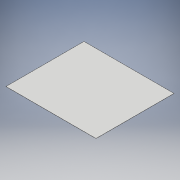
# Autodesk Inventor part: leftPanel
Saved by Autodesk Inventor 2017 (Build 210142000, 142)
## iProperties
Created: 2017-06-07
Part Number: leftPanel
Material: Generic
Document SubType Name: Sheet Metal
Designer: Roko
Density: 1 g/cm^3
Sheet Metal Rule: Default_mm
Appearance: Default
Author: Roko
Autodesk Inventor part; units mm, degrees
ref_plane "YZ Plane" through (0, 0, 0) normal (1, 0, 0) x (0, 1, 0)
ref_plane "XZ Plane" through (0, 0, 0) normal (0, 1, 0) x (-1, 0, 0)
ref_plane "XY Plane" through (0, 0, 0) normal (0, 0, 1) x (1, 0, 0)
sketch "Sketch1" plane through (0, 0, 0) normal (0, 0, 1) x (1, 0, 0)
  line L0 (-150, -130) -> (150, -130)
  line L1 (150, -130) -> (150, 130)
  line L2 (150, 130) -> (-150, 130)
  line L3 (-150, 130) -> (-150, -130)
  line L4 (-150, -130) -> (150, 130) construction
  line L5 (150, -130) -> (-150, 130) construction
  point P0 (0, 0)
  dimension "d0" = 300
  dimension "d1" = 260
  measures "d0" distance of L2.end L1.end
  measures "d1" distance of L1.end L0.end
extrude "Plate1" add sketch "Sketch1" along normal blind 0.5
equation "\"BendRadius\" = Thickness"
equation "\"BendReliefWidth\" = Thickness"
equation "\"BendReliefDepth\" = 0.5 * Thickness"
equation "\"CornerReliefSize\" = 4 * Thickness"
equation "\"MinimumRemnant\" = 2 * Thickness"
equation "\"TransitionRadius\" = BendRadius"
equation "\"JacobiRadiusSize\" = BendRadius"
equation "\"GapSize\" = Thickness"
equation "\"d2\" = BendRadius"
equation "\"Thickness\" = 0.5"
body "Solid1"
